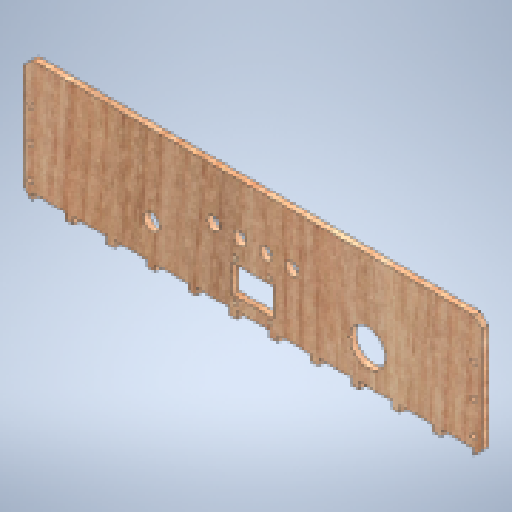
# Autodesk Inventor part: креп_мотора
Saved by Autodesk Inventor 2023.1 (Build 271208000, 208)
## iProperties
Created: 2025-12-22
Part Number: креп_мотора
Material: Древесина (береза)
Document SubType Name: Modeling
Designer: DELL
Density: 0.55 g/cm^3
Appearance: Береза — натуральный — полированный
Author: DELL
Autodesk Inventor part; units mm, degrees
ref_plane "YZ Plane" through (0, 0, 0) normal (1, 0, 0) x (0, 1, 0)
ref_plane "XZ Plane" through (0, 0, 0) normal (0, 1, 0) x (-1, 0, 0)
ref_plane "XY Plane" through (0, 0, 0) normal (0, 0, 1) x (1, 0, 0)
sketch "Эскиз1" plane through (0, 0, 0) normal (0, 0, 1) x (1, 0, 0)
  circle A0 centre (20.65, -19.15) radius 1.75 projected
  circle A1 centre (20.65, 0.85) radius 1.75 projected
  circle A2 centre (20.65, 20.85) radius 1.75 projected
  circle A3 centre (-251.15, -19.15) radius 1.75 projected
  circle A4 centre (-251.15, 0.85) radius 1.75 projected
  circle A5 centre (-251.15, 20.85) radius 1.75 projected
  line L0 (-255.45, -29.15) -> (-246.85, -29.15) projected
  line L1 (-255.65, -29.15) -> (-255.65, 270.85) projected
  line L2 (25.15, 270.85) -> (25.15, -29.15) projected
  line L3 (25.15, -29.15) -> (-255.65, -29.15)
  line L4 (-255.65, -29.15) -> (-255.65, 45.35)
  line L5 (-255.65, 45.35) -> (25.15, 45.35)
  line L6 (25.15, 45.35) -> (25.15, -29.15)
  point P0 (25.15, 45.35)
  constraints: 8 end point, 2 parallel, 1 horizontal, 1 perpendicular, 1 point on line
extrude "Выдавливание1" add sketch "Эскиз1" along normal blind 4
sketch "Эскиз4" plane through (0, 0, 4) normal (0, 0, 1) x (1, 0, 0)
  circle A0 centre (-177.15, -2.65) radius 5 construction
  line L0 (-177.15, -2.65) -> (-177.15, -29.15) construction
  line L1 (-255.65, -29.15) -> (25.15, -29.15) construction
  circle A1 centre (-177.15, -4.15) radius 5
  point P0 (0, 0)
  dimension "d30" = 10
  dimension "d31" = 25
  constraints: 2 centre point, 2 end point, 2 point on line, 1 vertical
  measures "d30" diameter of A1
  measures "d31" distance from line of L1 A1.centre
extrude "Выдавливание4" cut sketch "Эскиз4" against normal blind 10
sketch "Эскиз5" plane through (0, 0, 4) normal (0, 0, 1) x (1, 0, 0)
  line L0 (-127.9, -12.65) -> (-102.6, -12.65)
  line L1 (-102.6, -12.65) -> (-102.6, 4.35)
  line L2 (-102.6, 4.35) -> (-127.9, 4.35)
  line L3 (-127.9, 4.35) -> (-127.9, -12.65)
  line L4 (-127.9, -12.65) -> (-102.6, 4.35) construction
  line L5 (-102.6, -12.65) -> (-127.9, 4.35) construction
  circle A0 centre (-125.9, -15.9) radius 1.35
  line L6 (-115.25, -4.15) -> (-115.25, 2.5103)
  line L7 (-115.25, -4.15) -> (-117.239, -4.15)
  circle A1 centre (-104.6, -15.9) radius 1.35
  circle A2 centre (-125.9, 7.6) radius 1.35
  circle A3 centre (-104.6, 7.6) radius 1.35
  line L8 (-255.65, -29.15) -> (25.15, -29.15) projected
  line L9 (-115.25, -29.15) -> (-115.25, -2.4897) construction
  point P0 (0, 0)
  dimension "d33" = 17
  dimension "d39" = 2.7
  dimension "d40" = 3.25
  dimension "d41" = 2
  dimension "d45" = 25.3
  dimension "d46" = 25
  constraints: 18 end point, 4 centre point, 3 midpoint, 3 symmetric about line, 2 parallel, 1 horizontal, 1 perpendicular, 1 point on line, 1 vertical, 3 other
  measures "d33" distance of L1.end L0.end
  measures "d39" diameter of A0
  measures "d40" distance from line of L0 A0.centre
  measures "d41" distance from line of L3 A0.centre
  measures "d45" distance between parallel lines of L1 L3
  measures "d46" distance from line of L8 L6.start
extrude "Выдавливание5" cut sketch "Эскиз5" against normal blind 10
sketch "Эскиз6" plane through (0, 0, 4) normal (0, 0, 1) x (1, 0, 0)
  line L0 (-127.9, -12.65) -> (-127.9, 4.35) construction
  line L1 (-101.8454, -4.15) -> (-167.9603, -4.15) construction
  circle A0 centre (-44.85, -4.15) radius 11
  line L2 (-255.65, -29.15) -> (25.15, -29.15) projected
  circle A1 centre (-91.25, 19.35) radius 3.95
  line L3 (-127.9, 4.35) -> (-102.6, 4.35) projected
  line L4 (-102.6, 4.35) -> (-102.6, -12.65) projected
  line L5 (-91.25, 19.35) -> (-139.25, 19.35) construction
  line L6 (-115.25, 4.35) -> (-115.25, 38.684) construction
  circle A2 centre (-107.25, 19.35) radius 3.95
  circle A3 centre (-123.25, 19.35) radius 3.95
  circle A4 centre (-139.25, 19.35) radius 3.95
  line L7 (25.15, -29.15) -> (25.15, 45.35) projected
  point P0 (0, 0)
  point P1 (-127.9, -4.15)
  point P2 (-115.25, 19.35)
  dimension "d54" = 22
  dimension "d59" = 25
  dimension "d61" = 7.9
  dimension "d62" = 15
  dimension "d67" = 16
  dimension "d72" = 70
  constraints: 6 end point, 5 centre point, 3 horizontal, 3 midpoint, 2 point on line, 1 coincident, 1 vertical, 6 other
  measures "d54" diameter of A0
  measures "d59" distance from line of L2 A0.centre
  measures "d61" diameter of A1
  measures "d62" distance from line of L3 L5.start
  measures "d67" distance of L5.start A2.centre
  measures "d72" distance from line of L7 A0.centre
extrude "Выдавливание6" cut sketch "Эскиз6" against normal blind 10
chamfer "Фаска1" distance 5 angle 45 4 edges at (25.15, 45.35, 2) (-255.65, 45.35, 2) (-255.65, -29.15, 2) (25.15, -29.15, 2)
sketch "Эскиз7" plane through (0, 0, 4) normal (0, 0, 1) x (1, 0, 0)
  line L0 (-100.85, -29.15) -> (-100.85, -25.15)
  line L1 (-100.85, -25.15) -> (-84.85, -25.15)
  line L2 (-84.85, -25.15) -> (-84.85, -29.15)
  line L3 (-84.85, -29.15) -> (-100.85, -29.15)
  line L4 (-48.85, -29.15) -> (-48.85, -25.15)
  line L5 (-48.85, -25.15) -> (-32.85, -25.15)
  line L6 (-32.85, -25.15) -> (-32.85, -29.15)
  line L7 (-32.85, -29.15) -> (-48.85, -29.15)
  line L8 (19.15, -25.15) -> (19.15, -29.15)
  line L9 (19.15, -29.15) -> (3.15, -29.15)
  line L10 (3.15, -29.15) -> (3.15, -25.15)
  line L11 (3.15, -25.15) -> (19.15, -25.15)
  line L12 (-204.85, -29.15) -> (-204.85, -25.15)
  line L13 (-204.85, -25.15) -> (-188.85, -25.15)
  line L14 (-188.85, -25.15) -> (-188.85, -29.15)
  line L15 (-188.85, -29.15) -> (-204.85, -29.15)
  line L16 (-152.85, -29.15) -> (-152.85, -25.15)
  line L17 (-152.85, -25.15) -> (-136.85, -25.15)
  line L18 (-136.85, -25.15) -> (-136.85, -29.15)
  line L19 (-136.85, -29.15) -> (-152.85, -29.15)
  line L20 (-126.85, -29.15) -> (-126.85, -25.15)
  line L21 (-126.85, -25.15) -> (-110.85, -25.15)
  line L22 (-110.85, -25.15) -> (-110.85, -29.15)
  line L23 (-110.85, -29.15) -> (-126.85, -29.15)
  line L24 (-178.85, -29.15) -> (-178.85, -25.15)
  line L25 (-178.85, -25.15) -> (-162.85, -25.15)
  line L26 (-162.85, -25.15) -> (-162.85, -29.15)
  line L27 (-162.85, -29.15) -> (-178.85, -29.15)
  line L28 (-230.85, -29.15) -> (-230.85, -25.15)
  line L29 (-230.85, -25.15) -> (-214.85, -25.15)
  line L30 (-214.85, -25.15) -> (-214.85, -29.15)
  line L31 (-214.85, -29.15) -> (-230.85, -29.15)
  line L32 (-6.85, -25.15) -> (-6.85, -29.15)
  line L33 (-6.85, -29.15) -> (-22.85, -29.15)
  line L34 (-22.85, -29.15) -> (-22.85, -25.15)
  line L35 (-22.85, -25.15) -> (-6.85, -25.15)
  line L36 (-74.85, -29.15) -> (-74.85, -25.15)
  line L37 (-74.85, -25.15) -> (-58.85, -25.15)
  line L38 (-58.85, -25.15) -> (-58.85, -29.15)
  line L39 (-58.85, -29.15) -> (-74.85, -29.15)
  line L40 (-249.65, -29.15) -> (-249.65, -25.15)
  line L41 (-249.65, -25.15) -> (-236.85, -25.15)
  line L42 (-236.85, -25.15) -> (-236.85, -29.15)
  line L43 (-236.85, -29.15) -> (-249.65, -29.15)
  constraints: 88 end point, 22 horizontal, 22 vertical, 44 other
extrude "Выдавливание7" cut sketch "Эскиз7" against normal blind 4
sketch "Эскиз8" plane through (0, 0, 4) normal (0, 0, 1) x (1, 0, 0)
  line L0 (-32.85, -25.15) -> (-48.85, -25.15) construction
  line L1 (-48.85, -25.15) -> (-58.9685, -29.0911) construction
  circle A0 centre (-53.9092, -27.1206) radius 1.65
  line L2 (-162.85, -25.15) -> (-178.85, -25.15) construction
  line L3 (-188.85, -29.15) -> (-178.85, -29.15) construction
  line L4 (-178.85, -25.15) -> (-188.85, -29.15) construction
  circle A1 centre (-183.85, -27.15) radius 1.65
  point P0 (0, 0)
  dimension "d75" = 3.3
  dimension "d76" = 3.3
  constraints: 4 end point, 2 centre point, 2 midpoint
  measures "d75" diameter of A0
  measures "d76" diameter of A1
extrude "Выдавливание8" cut sketch "Эскиз8" against normal blind 4
